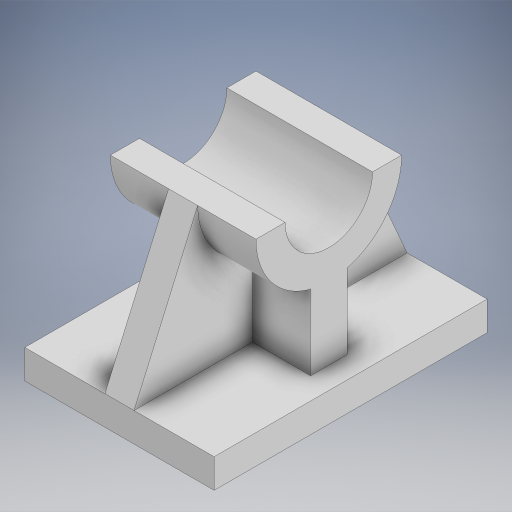
# Autodesk Inventor part: CE-1.3.3
Saved by Autodesk Inventor 2024 (Build 280153000, 153)
## iProperties
Created: 2024-01-25
Part Number: CE-1.3.3
Material: Generic
Document SubType Name: Modeling
Designer: Alex
Density: 1 g/cm^3
Appearance: Default
Author: Alex
Autodesk Inventor part; units mm, degrees
ref_plane "YZ Plane" through (0, 0, 0) normal (1, 0, 0) x (0, 1, 0)
ref_plane "XZ Plane" through (0, 0, 0) normal (0, 1, 0) x (-1, 0, 0)
sketch "Sketch1" plane through (0, 0, 0) normal (0, 1, 0) x (-1, 0, 0)
  line L0 (0, 0) -> (52, 0)
  line L1 (52, 0) -> (52, -75)
  line L2 (52, -75) -> (0, -75)
  line L3 (0, -75) -> (0, 0)
  dimension "d0" = 52
  dimension "d1" = 75
  constraints: 8 end point, 2 parallel, 1 horizontal, 1 perpendicular
  measures "d0" distance of L1.end L2.end
  measures "d1" distance of L0.end L1.end
extrude "Extrusion1" add sketch "Sketch1" along normal blind 8
ref_plane "Work Plane1" through (-6, 0, 0) normal (1, 0, 0) x (0, 0, -1)
sketch "Sketch4" plane through (-6, 0, 0) normal (1, 0, 0) x (0, 0, -1)
  line L0 (75, 0) -> (75, 8) projected
  line L1 (75, 8) -> (0, 8) projected
  line L2 (75, 0) -> (0, 0) projected
  line L3 (0, 0) -> (0, 8) projected
  line L4 (0, 0) -> (0, 8) construction
  line L5 (0, 8) -> (75, 8) construction
  line L6 (75, 0) -> (75, 8) construction
  line L7 (0, 0) -> (75, 0) construction
  line L8 (0, 0) -> (75, 0) projected
  line L9 (75, 0) -> (0, 0) projected
  line L10 (75, 8) -> (0, 8) projected
  line L11 (0, 8) -> (75, 8) projected
  line L12 (75, 0) -> (75, 8) projected
  line L13 (75, 0) -> (75, 8) projected
  line L14 (75, 0) -> (0, 0) projected
  line L15 (0, 0) -> (0, 8) projected
  line L16 (75, 8) -> (0, 8) projected
  line L17 (75, 0) -> (75, 8) projected
  line L18 (0, 0) -> (0, 8) projected
  line L19 (0, 0) -> (0, 8) projected
  line L20 (0, 0) -> (75, 0) projected
  line L21 (75, 0) -> (75, 8) projected
  line L22 (0, 8) -> (75, 8) projected
  line L23 (0, 0) -> (0, 8) projected
  line L24 (37.5, 8) -> (37.5, 48) construction
  arc A0 (25.5, 48) -> (49.5, 48) centre (37.5, 48) ccw
  line L25 (49.5, 48) -> (57.5, 48)
  line L26 (25.5, 48) -> (17.5, 48)
  line L27 (42.5, 8) -> (42.5, 28.6351)
  line L28 (32.5, 8) -> (32.5, 28.6351)
  arc A1 (17.5, 48) -> (32.5, 28.6351) centre (37.5, 48) ccw
  arc A2 (42.5, 28.6351) -> (57.5, 48) centre (37.5, 48) ccw
  dimension "d12" = 40
  dimension "d13" = 24
  dimension "d15" = 90
  dimension "d16" = 40
  dimension "d17" = 10
  dimension "d18" = 5
  dimension "d19" = 20
  dimension "d20" = 20
  constraints: 10 end point, 6 point on circle, 3 centre point, 3 point on line, 2 coincident, 2 parallel, 1 horizontal, 1 midpoint, 1 vertical
  measures "d12" distance of L24.start L24.end
  measures "d13" diameter of A0
  measures "d15" angle of L0 L26
  measures "d16" distance between parallel lines of L1 L25
  measures "d17" distance between parallel lines of L27 L28
  measures "d18" distance between parallel lines of L24 L27
  measures "d19" radius of A2
  measures "d20" radius of A1
extrude "Extrusion3" add sketch "Sketch4" against normal blind 40 contours L1 L28 A1 L26 A0 L25 A2 L27
ref_plane "Work Plane2" through (-22, 0, 0) normal (1, 0, 0) x (0, 0, -1)
sketch "Sketch5" plane through (-22, 0, 0) normal (1, 0, 0) x (0, 0, -1)
  line L0 (32.5, 8) -> (32.5, 28.6351) projected
  arc A0 (17.5, 48) -> (32.5, 28.6351) centre (37.5, 48) ccw projected
  line L1 (17.5, 48) -> (25.5, 48) construction
  arc A1 (25.5, 48) -> (49.5, 48) centre (37.5, 48) ccw construction
  line L2 (49.5, 48) -> (57.5, 48) construction
  arc A2 (42.5, 28.6351) -> (57.5, 48) centre (37.5, 48) ccw projected
  line L3 (42.5, 28.6351) -> (42.5, 8) projected
  line L4 (32.5, 8) -> (42.5, 8) construction
  line L5 (75, 8) -> (0, 8) projected
  line L6 (57.5, 48) -> (75, 8)
  line L7 (75, 8) -> (42.5, 8)
  line L8 (17.5, 48) -> (0, 8)
  line L9 (0, 8) -> (32.5, 8)
  point P0 (0, 0)
  constraints: 8 end point, 1 collinear, 1 perpendicular
extrude "Extrusion4" add sketch "Sketch5" against normal blind 8
body "Solid1"
